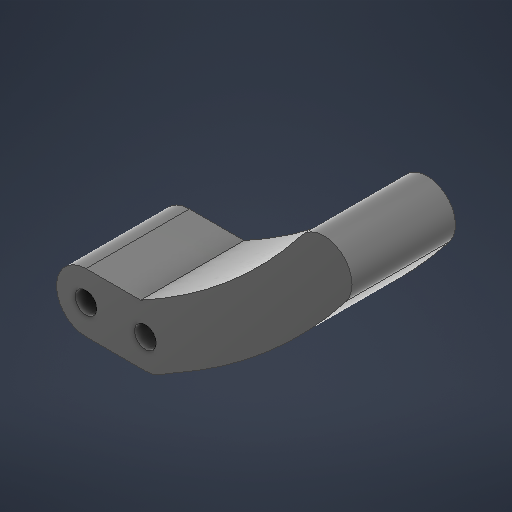
# Autodesk Inventor part: Lady Brown Ring Stop
Saved by Autodesk Inventor 2025 (Build 290162000, 162)
## iProperties
Created: 2024-12-29
Part Number: Lady Brown Ring Stop
Material: Generic
Document SubType Name: Modeling
Designer: Juan
Density: 1 g/cm^3
Appearance: Default
Author: Juan
Autodesk Inventor part; units mm, degrees
ref_plane "YZ Plane" through (0, 0, 0) normal (1, 0, 0) x (0, 1, 0)
ref_plane "XZ Plane" through (0, 0, 0) normal (0, 1, 0) x (-1, 0, 0)
ref_plane "XY Plane" through (0, 0, 0) normal (0, 0, 1) x (1, 0, 0)
sketch "Sketch1" plane through (0, 0, 0) normal (0, 0, 1) x (1, 0, 0)
  circle A0 centre (0, 0) radius 2.3241
  line L0 (0, 0) -> (12.7, 0) construction
  line L1 (0, -6.2992) -> (12.7, -6.2992)
  line L2 (12.7, 6.2992) -> (0, 6.2992)
  arc A1 (0, 6.2992) -> (0, -6.2992) centre (0, 0) ccw
  arc A2 (12.7, -6.2992) -> (12.7, 6.2992) centre (12.7, 0) ccw
  line L3 (12.7, 0) -> (50.8, 0)
  line L4 (50.8, 0) -> (50.8, 31.75)
  arc A3 (12.7, 0) -> (50.8, 31.75) centre (-39.6067, 101.5031) ccw
  line L5 (12.7, 0) -> (12.7, 6.2992)
  line L6 (12.7, -6.2992) -> (12.7, 0)
  arc A4 (12.7, 0) -> (50.8, 31.75) centre (-39.6067, 101.5031) ccw construction
  arc A5 (15.4698, -5.3749) -> (55.5873, 28.0564) centre (-39.6067, 101.5031) ccw
  arc A6 (9.9302, 5.3749) -> (46.0127, 35.4436) centre (-39.6067, 101.5031) ccw
  arc A7 (9.9302, 5.3749) -> (15.4698, -5.3749) centre (12.7, 0) ccw
  arc A8 (55.5873, 28.0564) -> (46.0127, 35.4436) centre (50.8, 31.75) ccw
  circle A9 centre (12.7, 0) radius 2.3241
  point P0 (6.35, 0)
  point P1 (17.0744, -4.5326)
  point P2 (11.6843, 6.2992)
  dimension "d0" = 4.6482
  dimension "d1" = 12.7
  dimension "d2" = 12.5984
  dimension "d3" = 38.1
  dimension "d4" = 31.75
  dimension "d5" = 4.6482
  constraints: 16 end point, 16 point on circle, 10 centre point, 8 tangent, 2 coincident, 2 equal length, 2 horizontal, 2 perpendicular, 1 concentric, 1 midpoint
  measures "d0" diameter of A0
  measures "d1" distance of L0.start L0.end
  measures "d2" diameter of A2
  measures "d3" distance of L0.end L3.end
  measures "d4" distance of L3.end L4.end
  measures "d5" diameter of A9
extrude "Extrusion1" add sketch "Sketch1" along normal blind 22.098 contours A1 L2 A6 A7 L6 L1 | L6 A7 A5 A2 | A5 A7 L6 A9 L3 A2 | A2 L3 A5 | A7 A6 L2 L5 A9 L6 | A6 A8 A5 L4 A3 A2 L2 | L3 A9 A3 A2 | A2 A3 L4 A5 L3 | A2 A3 A9 L5
fillet "Fillet1" radius 25.4 1 edges at (17.0744, -4.5326, 11.049)
body "Solid1"
